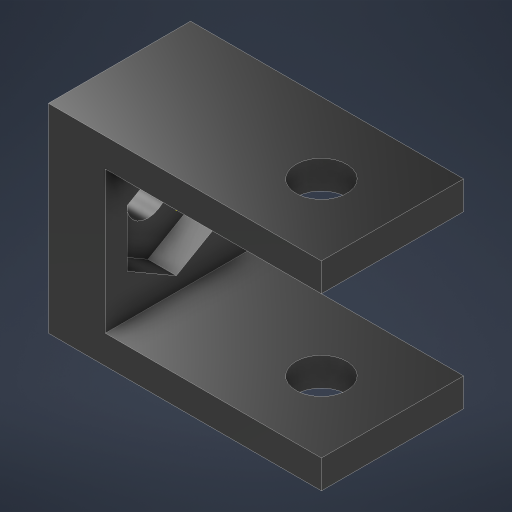
# Autodesk Inventor part: printed piston fitting wings
Saved by Autodesk Inventor 2024 (Build 280153000, 153)
## iProperties
Created: 2024-02-08
Part Number: printed piston fitting wings
Material: Generic
Document SubType Name: Modeling
Designer: elite
Density: 1 g/cm^3
Appearance: Glossy - Black
Author: elite
Autodesk Inventor part; units mm, degrees
ref_plane "YZ Plane" through (0, 0, 0) normal (1, 0, 0) x (0, 1, 0)
ref_plane "XZ Plane" through (0, 0, 0) normal (0, 1, 0) x (-1, 0, 0)
ref_plane "XY Plane" through (0, 0, 0) normal (0, 0, 1) x (1, 0, 0)
sketch "Sketch1" plane through (0, 0, 0) normal (1, 0, 0) x (0, 1, 0)
  circle A0 centre (0, 0) radius 1.905
  line L0 (0, 0) -> (0, -6.35)
  line L1 (0, 0) -> (0, 6.35)
  line L2 (0, 6.35) -> (-6.35, 6.35)
  line L3 (0, -6.35) -> (6.35, -6.35)
  line L4 (-6.35, 6.35) -> (6.35, 6.35)
  line L5 (6.35, 6.35) -> (6.35, -6.35)
  line L6 (6.35, -6.35) -> (-6.35, -6.35)
  line L7 (-6.35, -6.35) -> (-6.35, 6.35)
  dimension "d0" = 3.81
  dimension "d2" = 6.35
  dimension "d3" = 6.35
  dimension "d4" = 6.35
  dimension "d5" = 6.35
  constraints: 16 end point, 3 horizontal, 2 parallel, 2 vertical, 1 centre point, 1 coincident, 1 perpendicular
  measures "d0" diameter of A0
  measures "d2" distance of L0.start L0.end
  measures "d3" distance of L0.start L1.end
  measures "d4" distance of L1.end L2.end
  measures "d5" distance of L0.end L3.end
extrude "Extrusion1" add sketch "Sketch1" along normal blind 5.08 contours A0 L1 L4 L5 L3 L0 | A0 L0 L6 L7 L2 L1
sketch "Sketch2" plane through (5.08, 0, 0) normal (1, 0, 0) x (0, 0, -1)
  point P0 (0, 0)
sketch "Sketch3" plane through (5.08, 0, 0) normal (1, 0, 0) x (0, 0, -1)
  line L0 (0, 0) -> (0, -5.08)
  arc A0 (0, -5.08) -> (0, 0) centre (-4.3994, -2.54) ccw
  line L1 (4.3994, -2.54) -> (0, -5.08)
  line L2 (0, -5.08) -> (-4.3994, -2.54)
  line L3 (-4.3994, 2.54) -> (0, 5.08)
  line L4 (4.3994, 2.54) -> (4.3994, -2.54)
  line L5 (-4.3994, -2.54) -> (-4.3994, 2.54)
  line L6 (0, 5.08) -> (4.3994, 2.54)
  dimension "d8" = 5.08
  constraints: 14 end point, 3 vertical, 2 point on circle, 1 centre point, 1 parallel
  measures "d8" distance of L0.end L0.start
extrude "Extrusion2" cut sketch "Sketch3" against normal blind 2.54 contours A0 L0 | L2 L5 L3 L6 L4 L1
sketch "Sketch4" plane through (0, -6.35, -6.35) normal (0, -1, 0) x (1, 0, 0)
  line L0 (0, 12.7) -> (5.08, 12.7) projected
  line L1 (0, 0) -> (5.08, 0) projected
  line L2 (5.08, 12.7) -> (0, 12.7)
  line L3 (0, 12.7) -> (0, 0)
  line L4 (0, 0) -> (5.08, 0)
  line L5 (5.08, 0) -> (5.08, 12.7)
  point P0 (0, 6.35)
  constraints: 8 end point, 2 parallel, 1 horizontal, 1 perpendicular
extrude "Extrusion3" add sketch "Sketch4" along normal blind 2.54
sketch "Sketch5" plane through (0, 6.35, 6.35) normal (0, 1, 0) x (1, 0, 0)
  line L0 (5.08, 0) -> (0, 0) projected
  line L1 (5.08, 12.7) -> (5.08, 0) projected
  line L2 (0, 0) -> (5.08, 0)
  line L3 (5.08, 0) -> (5.08, 12.7)
  line L4 (5.08, 12.7) -> (0, 12.7)
  line L5 (0, 12.7) -> (0, 0)
  point P0 (0, 6.35)
  constraints: 8 end point, 2 parallel, 1 horizontal, 1 perpendicular
extrude "Extrusion4" add sketch "Sketch5" along normal blind 2.54
sketch "Sketch6" plane through (5.08, 0, 0) normal (1, 0, 0) x (0, 0, -1)
  line L0 (-6.35, -8.89) -> (-6.35, 8.89) projected
  line L1 (-6.35, 8.89) -> (-6.35, 6.35)
  line L2 (-6.35, -8.89) -> (-6.35, -6.35)
  line L3 (6.35, 8.89) -> (-6.35, 8.89) projected
  line L4 (-6.35, 6.35) -> (6.35, 6.35)
  line L5 (6.35, 6.35) -> (6.35, 8.89)
  line L6 (6.35, 8.89) -> (-6.35, 8.89)
  line L7 (-6.35, 8.89) -> (-6.35, 6.35)
  line L8 (6.35, -8.89) -> (-6.35, -8.89) projected
  line L9 (-6.35, -6.35) -> (6.35, -6.35)
  line L10 (6.35, -6.35) -> (6.35, -8.89)
  line L11 (6.35, -8.89) -> (-6.35, -8.89)
  line L12 (-6.35, -8.89) -> (-6.35, -6.35)
  point P0 (0, 0)
  dimension "d15" = 2.54
  dimension "d16" = 2.54
  constraints: 20 end point, 4 parallel, 2 horizontal, 2 perpendicular, 2 point on line
  measures "d15" distance of L0.end L1.end
  measures "d16" distance of L0.start L2.end
extrude "Extrusion5" add sketch "Sketch6" along normal blind 19.304
sketch "Sketch7" plane through (0, -8.89, -6.35) normal (0, -1, 0) x (1, 0, 0)
  line L0 (24.384, 0) -> (24.384, 12.7) projected
  line L1 (24.384, 6.35) -> (18.034, 6.35)
  circle A0 centre (18.034, 6.35) radius 2.2606
  point P0 (0, 6.35)
  dimension "d19" = 6.35
  dimension "d20" = 4.5212
  constraints: 2 end point, 1 centre point, 1 coincident, 1 horizontal, 1 midpoint
  measures "d19" distance of L1.start L1.end
  measures "d20" diameter of A0
extrude "Extrusion6" cut sketch "Sketch7" against normal blind 63.5
body "Solid1"
